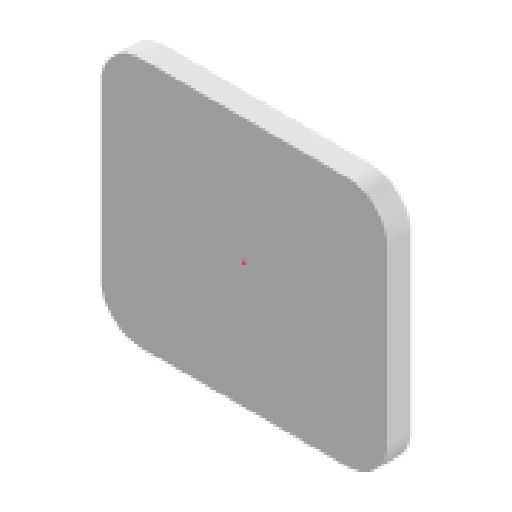
# Autodesk Inventor part: Display_black_cover
Saved by Autodesk Inventor 2025 (Build 290162000, 162)
## iProperties
Created: 2025-01-03
Part Number: Display_black_cover
Material: Generic
Document SubType Name: Modeling
Designer: Jan Mareš
Density: 1 g/cm^3
Appearance: Default
Author: Jan Mareš
Autodesk Inventor part; units mm, degrees
ref_plane "YZ Plane" through (0, 0, 0) normal (1, 0, 0) x (0, 1, 0)
ref_plane "XZ Plane" through (0, 0, 0) normal (0, 1, 0) x (-1, 0, 0)
ref_plane "XY Plane" through (0, 0, 0) normal (0, 0, 1) x (1, 0, 0)
sketch "Sketch1" plane through (0, 0, 0) normal (0, 0, 1) x (1, 0, 0)
  line L0 (0, -35) -> (0, 35) construction
  line L1 (-42, 0) -> (42, 0) construction
  line L2 (30, -25) -> (-30, -25)
  line L3 (-30, -25) -> (-30, 25)
  line L4 (-30, 25) -> (30, 25)
  line L5 (30, 25) -> (30, -25)
  line L6 (-30, 0) -> (30, 0) construction
  point P0 (0, 0)
  dimension "d0" = 60
  dimension "d1" = 50
  constraints: 10 end point, 3 midpoint, 2 parallel, 1 horizontal, 1 perpendicular
  measures "d0" distance of L3.end L4.end
  measures "d1" distance of L2.end L3.end
extrude "Extrusion1" add sketch "Sketch1" along normal mid plane 4
sketch "Sketch2" plane through (0, 0, -2) normal (0, 0, -1) x (-1, 0, 0)
  arc A0 (-21.5, -14.5) -> (-17.5, -18.5) centre (-17.5, -14.5) ccw construction
  line L0 (-21.5, 14.5) -> (-21.5, -14.5) construction
  arc A1 (-17.5, 18.5) -> (-21.5, 14.5) centre (-17.5, 14.5) ccw construction
  line L1 (17.5, 18.5) -> (-17.5, 18.5) construction
  arc A2 (21.5, 14.5) -> (17.5, 18.5) centre (17.5, 14.5) ccw construction
  line L2 (21.5, -14.5) -> (21.5, 14.5) construction
  arc A3 (17.5, -18.5) -> (21.5, -14.5) centre (17.5, -14.5) ccw construction
  line L3 (-17.5, -18.5) -> (17.5, -18.5) construction
  arc A4 (-24.3, -14.5) -> (-17.5, -21.3) centre (-17.5, -14.5) ccw
  line L4 (-17.5, -21.3) -> (17.5, -21.3)
  arc A5 (17.5, -21.3) -> (24.3, -14.5) centre (17.5, -14.5) ccw
  line L5 (24.3, -14.5) -> (24.3, 14.5)
  arc A6 (24.3, 14.5) -> (17.5, 21.3) centre (17.5, 14.5) ccw
  line L6 (17.5, 21.3) -> (-17.5, 21.3)
  arc A7 (-17.5, 21.3) -> (-24.3, 14.5) centre (-17.5, 14.5) ccw
  line L7 (-24.3, 14.5) -> (-24.3, -14.5)
  line L8 (-30, 25) -> (-30, -25) projected
  line L9 (30, 25) -> (-30, 25) projected
  line L10 (30, -25) -> (30, 25) projected
  line L11 (-30, -25) -> (30, -25) projected
  point P0 (0, 0)
  dimension "d4" = 2.8
  constraints: 8 end point, 8 point on circle, 4 centre point, 7 other
  measures "d4" distance between parallel lines of L0 L7
extrude "Extrusion2" cut sketch "Sketch2" against normal blind 10
sketch "Sketch5" plane through (0, 0, 2) normal (0, 0, 1) x (1, 0, 0)
  line L0 (22.6, -14.4) -> (22.6, 14.4) construction
  arc A0 (17.4, -19.6) -> (22.6, -14.4) centre (17.4, -14.4) ccw construction
  line L1 (-17.4, -19.6) -> (17.4, -19.6) construction
  arc A1 (-22.6, -14.4) -> (-17.4, -19.6) centre (-17.4, -14.4) ccw construction
  line L2 (-22.6, 14.4) -> (-22.6, -14.4) construction
  arc A2 (-17.4, 19.6) -> (-22.6, 14.4) centre (-17.4, 14.4) ccw construction
  line L3 (17.4, 19.6) -> (-17.4, 19.6) construction
  arc A3 (22.6, 14.4) -> (17.4, 19.6) centre (17.4, 14.4) ccw construction
  line L4 (22.7, 14.4) -> (22.7, -14.4)
  arc A4 (17.4, -19.7) -> (22.7, -14.4) centre (17.4, -14.4) ccw
  line L5 (17.4, -19.7) -> (-17.4, -19.7)
  arc A5 (-22.7, -14.4) -> (-17.4, -19.7) centre (-17.4, -14.4) ccw
  line L6 (-22.7, -14.4) -> (-22.7, 14.4)
  arc A6 (-17.4, 19.7) -> (-22.7, 14.4) centre (-17.4, 14.4) ccw
  line L7 (-17.4, 19.7) -> (17.4, 19.7)
  arc A7 (22.7, 14.4) -> (17.4, 19.7) centre (17.4, 14.4) ccw
  point P0 (0, 0)
  dimension "d7" = 0.1
  constraints: 8 end point, 8 point on circle, 4 centre point, 7 other
  measures "d7" distance between parallel lines of L0 L4
extrude "Extrusion3" cut sketch "Sketch5" against normal blind 3.3
sketch "Sketch6" plane through (0, 0, 2) normal (0, 0, 1) x (1, 0, 0)
  line L0 (-23.7, 14.5) -> (-23.7, -14.5) construction
  arc A0 (-17.5, 20.7) -> (-23.7, 14.5) centre (-17.5, 14.5) ccw construction
  line L1 (17.5, 20.7) -> (-17.5, 20.7) construction
  arc A1 (23.7, 14.5) -> (17.5, 20.7) centre (17.5, 14.5) ccw construction
  line L2 (23.7, -14.5) -> (23.7, 14.5) construction
  arc A2 (17.5, -20.7) -> (23.7, -14.5) centre (17.5, -14.5) ccw construction
  line L3 (-17.5, -20.7) -> (17.5, -20.7) construction
  arc A3 (-23.7, -14.5) -> (-17.5, -20.7) centre (-17.5, -14.5) ccw construction
  arc A4 (17.5, -20.7) -> (23.7, -14.5) centre (17.5, -14.5) ccw construction
  arc A5 (23.55, 14.5) -> (17.5, 20.55) centre (17.5, 14.5) ccw
  line L4 (17.5, 20.55) -> (-17.5, 20.55)
  arc A6 (-17.5, 20.55) -> (-23.55, 14.5) centre (-17.5, 14.5) ccw
  line L5 (-23.55, 14.5) -> (-23.55, -14.5)
  arc A7 (-23.55, -14.5) -> (-17.5, -20.55) centre (-17.5, -14.5) ccw
  line L6 (-17.5, -20.55) -> (17.5, -20.55)
  arc A8 (17.5, -20.55) -> (23.55, -14.5) centre (17.5, -14.5) ccw
  line L7 (23.55, -14.5) -> (23.55, 14.5)
  arc A9 (27.7, 14.5) -> (17.5, 24.7) centre (17.5, 14.5) ccw
  line L8 (17.5, 24.7) -> (-17.5, 24.7)
  arc A10 (-17.5, 24.7) -> (-27.7, 14.5) centre (-17.5, 14.5) ccw
  line L9 (-27.7, 14.5) -> (-27.7, -14.5)
  arc A11 (-27.7, -14.5) -> (-17.5, -24.7) centre (-17.5, -14.5) ccw
  line L10 (-17.5, -24.7) -> (17.5, -24.7)
  arc A12 (17.5, -24.7) -> (27.7, -14.5) centre (17.5, -14.5) ccw
  line L11 (27.7, -14.5) -> (27.7, 14.5)
  point P0 (0, 0)
  dimension "d14" = 0.15
  dimension "d15" = 4
  constraints: 16 end point, 16 point on circle, 8 centre point, 14 other
  measures "d14" distance between parallel lines of L2 L7
  measures "d15" distance between parallel lines of L2 L11
extrude "Extrusion4" cut sketch "Sketch6" against normal blind 2.1
sketch "Sketch7" plane through (0, 0, 0) normal (0, 1, 0) x (-1, 0, 0)
  line L0 (23.55, 2) -> (23.55, -0.1) construction
  line L1 (23.55, 1) -> (23.77, 0.4)
  line L2 (23.77, 0.4) -> (23.55, 0.4)
  line L3 (23.55, 1) -> (23.55, 0.4)
  line L4 (-17.5, 2) -> (-23.55, 2) construction
  line L5 (-23.55, 2) -> (-17.5, 2) construction
  line L6 (-17.5, 2) -> (17.5, 2) construction
  line L7 (17.5, 2) -> (23.55, 2) construction
  line L8 (23.55, 2) -> (17.5, 2) construction
  line L9 (17.5, 2) -> (-17.5, 2) construction
  line L10 (17.4, 2) -> (22.7, 2) construction
  line L11 (22.7, 2) -> (17.4, 2) construction
  line L12 (17.4, 2) -> (-17.4, 2) construction
  line L13 (-17.4, 2) -> (-22.7, 2) construction
  line L14 (-22.7, 2) -> (-17.4, 2) construction
  line L15 (-17.4, 2) -> (17.4, 2) construction
  point P0 (0, 0)
  dimension "d16" = 1.6
  dimension "d17" = 0.6
  dimension "d18" = 0.22
  constraints: 6 end point, 2 point on line, 1 collinear, 1 perpendicular
  measures "d16" distance between parallel lines of L2 L8
  measures "d17" distance of L1.start L2.end
  measures "d18" distance of L1.end L2.end
sketch "Sketch8" plane through (0, 0, 2) normal (0, 0, 1) x (1, 0, 0)
  line L0 (-23.55, 14.5) -> (-23.55, -14.5) projected
  arc A0 (-23.55, -14.5) -> (-17.5, -20.55) centre (-17.5, -14.5) ccw projected
  line L1 (-17.5, -20.55) -> (17.5, -20.55) projected
  arc A1 (17.5, -20.55) -> (23.55, -14.5) centre (17.5, -14.5) ccw projected
  line L2 (23.55, -14.5) -> (23.55, 14.5) projected
  arc A2 (23.55, 14.5) -> (17.5, 20.55) centre (17.5, 14.5) ccw projected
  line L3 (17.5, 20.55) -> (-17.5, 20.55) projected
  arc A3 (-17.5, 20.55) -> (-23.55, 14.5) centre (-17.5, 14.5) ccw projected
  point P0 (0, 0)
sketch3d "3D Sketch1"
  arc A0 (-23.55, -14.5, 2) -> (-17.5, -20.55, 2) centre (-17.5, -14.5, 2) ccw
  line L0 (-17.5, -20.55, 2) -> (17.5, -20.55, 2)
  arc A1 (17.5, -20.55, 2) -> (23.55, -14.5, 2) centre (17.5, -14.5, 2) ccw
  line L1 (23.55, -14.5, 2) -> (23.55, 14.5, 2)
  arc A2 (23.55, 14.5, 2) -> (17.5, 20.55, 2) centre (17.5, 14.5, 2) ccw
  line L2 (17.5, 20.55, 2) -> (-17.5, 20.55, 2)
  arc A3 (-17.5, 20.55, 2) -> (-23.55, 14.5, 2) centre (-17.5, 14.5, 2) ccw
  line L3 (-23.55, 14.5, 2) -> (-23.55, -14.5, 2)
sweep "Sweep1" add profiles "Sketch7" path "3D Sketch1"
fillet "Fillet1" radius 0.02 8 edges at (-21.9336, -18.9336, 0.4) (0, -20.77, 0.4) (21.9336, -18.9336, 0.4) (23.77, 0, 0.4) (21.9336, 18.9336, 0.4) (0, 20.77, 0.4) (-21.9336, 18.9336, 0.4) (-23.77, 0, 0.4)
sketch "Sketch9" plane through (0, 0, -1.3) normal (0, 0, 1) x (1, 0, 0)
  line L0 (18.5, 15.5) -> (-11.5, 15.5) construction
  line L1 (-11.5, 15.5) -> (-11.5, 1.5) construction
  line L2 (18.5, 1.5) -> (18.5, 15.5) construction
  line L3 (-11.5, 1.5) -> (18.5, 1.5) construction
  line L4 (18.5, -1.5) -> (-11.5, -1.5) construction
  line L5 (18.5, -15.5) -> (18.5, -1.5) construction
  line L6 (-11.5, -15.5) -> (18.5, -15.5) construction
  line L7 (-11.5, -1.5) -> (-11.5, -15.5) construction
  line L8 (-11.9, 1.1) -> (-11.9, 15.9)
  line L9 (-11.9, 15.9) -> (18.9, 15.9)
  line L10 (18.9, 15.9) -> (18.9, 1.1)
  line L11 (18.9, 1.1) -> (-11.9, 1.1)
  line L12 (-11.9, -15.9) -> (18.9, -15.9)
  line L13 (18.9, -15.9) -> (18.9, -1.1)
  line L14 (18.9, -1.1) -> (-11.9, -1.1)
  line L15 (-11.9, -1.1) -> (-11.9, -15.9)
  point P0 (0, 0)
  dimension "d22" = 0.4
  dimension "d23" = 0.4
  constraints: 16 end point, 6 other
  measures "d22" distance between parallel lines of L1 L8
  measures "d23" distance between parallel lines of L7 L15
extrude "Extrusion5" cut sketch "Sketch9" against normal through all
sketch "Sketch12" plane through (0, 0, -2) normal (0, 0, -1) x (-1, 0, 0)
  line L0 (-18.9, 1.1) -> (-18.9, 15.9) projected
  line L1 (-18.9, 15.9) -> (11.9, 15.9) projected
  line L2 (11.9, 15.9) -> (11.9, 1.1) projected
  line L3 (11.9, 1.1) -> (-18.9, 1.1) projected
  line L4 (-18.9, -1.1) -> (11.9, -1.1) projected
  line L5 (-18.9, -15.9) -> (-18.9, -1.1) projected
  line L6 (11.9, -15.9) -> (-18.9, -15.9) projected
  line L7 (11.9, -1.1) -> (11.9, -15.9) projected
  line L8 (-20.9, 17.9) -> (13.9, 17.9)
  line L9 (13.9, 17.9) -> (13.9, -17.9)
  line L10 (13.9, -17.9) -> (-20.9, -17.9)
  line L11 (-20.9, -17.9) -> (-20.9, 17.9)
  line L12 (-3.5, 15.9) -> (-3.5, 17.9) construction
  line L13 (11.9, 8.5) -> (13.9, 8.5) construction
  line L14 (-18.9, 8.5) -> (-20.9, 8.5) construction
  line L15 (-3.5, -15.9) -> (-3.5, -17.9) construction
  point P0 (0, 0)
  dimension "d35" = 2
  constraints: 16 end point, 7 midpoint, 7 perpendicular, 3 equal length, 2 point on line, 1 horizontal
  measures "d35" distance of point (-3.5, 15.9) L12.end
extrude "Extrusion6" add sketch "Sketch12" along normal blind 7
fillet "Fillet2" radius 2 4 edges at (20.9, 17.9, -5.5) (20.9, -17.9, -5.5) (-13.9, -17.9, -5.5) (-13.9, 17.9, -5.5)
body "Solid1"
